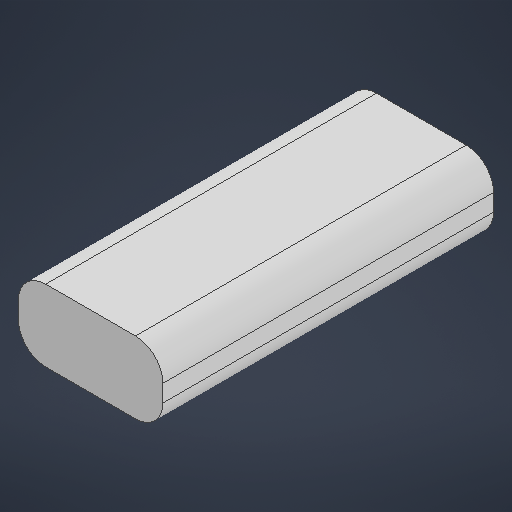
# Autodesk Inventor part: battery-model-group2
Saved by Autodesk Inventor 2026.1 (Build 301233000, 233)
## iProperties
Created: 2026-02-24
Part Number: battery-model-group2
Material: Generic
Document SubType Name: Modeling
Designer: aj2074
Density: 1 g/cm^3
Appearance: Default
Author: aj2074
Autodesk Inventor part; units mm, degrees
ref_plane "YZ Plane" through (0, 0, 0) normal (1, 0, 0) x (0, 1, 0)
ref_plane "XZ Plane" through (0, 0, 0) normal (0, 1, 0) x (-1, 0, 0)
ref_plane "XY Plane" through (0, 0, 0) normal (0, 0, 1) x (1, 0, 0)
sketch "Sketch1" plane through (0, 0, 0) normal (0, 1, 0) x (-1, 0, 0)
  line L0 (402.7378, 921.7891) -> (0, 921.7891)
  line L1 (0, 921.7891) -> (0, 0)
  line L2 (0, 0) -> (402.7378, 0)
  line L3 (402.7378, 0) -> (402.7378, 921.7891)
  constraints: 8 end point, 2 parallel, 1 horizontal, 1 perpendicular
extrude "Extrusion1" add sketch "Sketch1" along normal blind 200
fillet "Fillet1" radius 76.2 1 edges at (0, 200, 460.8945)
fillet "Fillet2" radius 76.2 1 edges at (0, 0, 460.8945)
fillet "Fillet3" radius 76.2 1 edges at (-402.7378, 200, 460.8945)
fillet "Fillet4" radius 76.2 1 edges at (-402.7378, 0, 460.8945)
